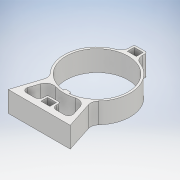
# Autodesk Inventor part: Motor Reversed Mount Midsection
Saved by Autodesk Inventor 2018 (Build 220112000, 112)
## iProperties
Created: 2018-01-25
Part Number: Motor Reversed Mount Midsection
Material: ABS Plastic
Document SubType Name: Modeling
Designer: Moochster
Density: 1.06 g/cm^3
Appearance: Smooth - White
Author: Moochster
Autodesk Inventor part; units mm, degrees
ref_plane "YZ Plane" through (0, 0, 0) normal (1, 0, 0) x (0, 1, 0)
ref_plane "XZ Plane" through (0, 0, 0) normal (0, 1, 0) x (-1, 0, 0)
ref_plane "XY Plane" through (0, 0, 0) normal (0, 0, 1) x (1, 0, 0)
sketch "Sketch1" plane through (0, 0, 0) normal (0, 0, 1) x (1, 0, 0)
  circle A0 centre (0, 0) radius 15.015
  circle A1 centre (0, 0) radius 16.015
  line L0 (-10, -12.5092) -> (-15, -28)
  line L1 (-15, -28) -> (15, -28)
  line L2 (15, -28) -> (10, -12.5092)
  line L3 (8.2846, -13.7057) -> (11.9301, -25)
  line L4 (11.9301, -25) -> (3.15, -25)
  line L5 (-11.9301, -25) -> (-8.2846, -13.7057)
  line L6 (-1.5, -14.9399) -> (-1.5, -14.515)
  line L7 (-1, -14.015) -> (1, -14.015)
  line L8 (1.5, -14.515) -> (1.5, -14.9399)
  arc A2 (-1, -14.015) -> (-1.5, -14.515) centre (-1, -14.515) ccw
  arc A3 (1.5, -14.515) -> (1, -14.015) centre (1, -14.515) ccw
  line L9 (2, -25) -> (2, -22) construction
  line L10 (2, -22) -> (-2, -22) construction
  line L11 (-2, -22) -> (-2, -25) construction
  line L12 (-2.15, -25) -> (-2.15, -21.85)
  line L13 (-2.15, -21.85) -> (2.15, -21.85)
  line L14 (2.15, -21.85) -> (2.15, -25)
  line L15 (-3.15, -25) -> (-3.15, -20.85)
  line L16 (-3.15, -20.85) -> (3.15, -20.85)
  line L17 (3.15, -20.85) -> (3.15, -25)
  line L18 (3.15, -25) -> (2.15, -25)
  line L19 (2.15, -25) -> (-2.15, -25)
  line L20 (-2.15, -25) -> (-3.15, -25)
  line L21 (-3.15, -25) -> (-11.9301, -25)
  line L22 (2, 20) -> (-2, 20) construction
  line L23 (-2, 20) -> (-2, 17) construction
  line L24 (-2, 17) -> (2, 17) construction
  line L25 (2, 17) -> (2, 20) construction
  line L26 (-2.15, 16.85) -> (-2.15, 20.15)
  line L27 (-2.15, 20.15) -> (2.15, 20.15)
  line L28 (2.15, 20.15) -> (2.15, 16.85)
  line L29 (2.15, 16.85) -> (-2.15, 16.85)
  line L30 (3.15, 15.7022) -> (3.15, 21.15)
  line L31 (3.15, 21.15) -> (-3.15, 21.15)
  line L32 (-3.15, 21.15) -> (-3.15, 15.7022)
  point P0 (0, -28)
  point P1 (-1.5, -14.015)
  point P2 (1.5, -14.015)
  point P3 (0, -14.015)
  point P4 (0, -15.015)
  point P5 (0, -22)
  point P6 (0, -25)
  point P7 (0, -25)
  point P8 (0, 17)
  dimension "d0" = 28
  dimension "d1" = 1
  dimension "d2" = 30
  dimension "d3" = 30.03
  dimension "d4" = 20
  dimension "d5" = 3
  dimension "d6" = 2
  dimension "d10" = 3
  dimension "d12" = 1
  dimension "d13" = 0.5
  dimension "d14" = 3
  dimension "d15" = 4
  dimension "d16" = 0.15
  dimension "d17" = 1
  dimension "d21" = 4
  dimension "d22" = 3
  dimension "d23" = 17
  dimension "d24" = 0.15
  dimension "d25" = 1
  dimension "d26" = 1
  dimension "d27" = 1
  constraints: 66 end point, 13 point on circle, 12 perpendicular, 10 point on line, 7 vertical alignment, 5 midpoint, 4 centre point, 4 parallel, 4 tangent, 4 vertical, 3 horizontal, 2 coincident, 2 horizontal alignment, 1 equal length, 1 equal radius, 7 other
  measures "d0" distance from line of point (0, 0) L1
  measures "d1" radial gap between concentric circles of A1 A0
  measures "d2" distance of L0.end L1.end
  measures "d3" diameter of A0
  measures "d4" distance of L0.start L2.end
  measures "d5" distance between parallel lines of L1 L4
  measures "d6" distance between parallel lines of L2 L3
  measures "d10" distance of point (-1.5, -14.015) point (1.5, -14.015)
  measures "d12" distance from line of L7 point (0, -15.015)
  measures "d13" radius of A2
  measures "d14" distance of L10.end L11.end
  measures "d15" distance of L9.end L10.end
  measures "d16" distance between parallel lines of L11 L12
  measures "d17" distance between parallel lines of L12 L15
  measures "d21" distance of L22.start L22.end
  measures "d22" distance of L22.end L23.end
  measures "d23" distance from line of A0.centre L24
  measures "d24" distance between parallel lines of L26 L23
  measures "d25" distance between parallel lines of L26 L32
  measures "d26" distance between parallel lines of L30 L28
  measures "d27" distance between parallel lines of L27 L31
extrude "Extrusion1" add sketch "Sketch1" along normal blind 10 contours L6 A2 L7 A3 L8 A0 | A1 | A1 L32 L31 L30 | L2 L1 L0 A1 L5 L21 L20 L19 L18 L4 L3 | L18 L14 L13 L12 L20 L15 L16 L17 picked at (0.1669, -14.3455)
fillet "Fillet1" radius 4 6 edges at (10, -12.5092, 5) (8.2846, -13.7057, 5) (-8.2846, -13.7057, 5) (-10, -12.5092, 5) (3.15, 15.7022, 5) (-3.15, 15.7022, 5)
fillet "Fillet1" radius 2 4 edges at (11.9301, -25, 5) (-11.9301, -25, 5) (-3.15, -25, 5) (3.15, -25, 5)
fillet "Fillet1" radius 1 4 edges at (3.15, -20.85, 5) (-3.15, -20.85, 5) (3.15, 21.15, 5) (-3.15, 21.15, 5)
body "Solid1"
